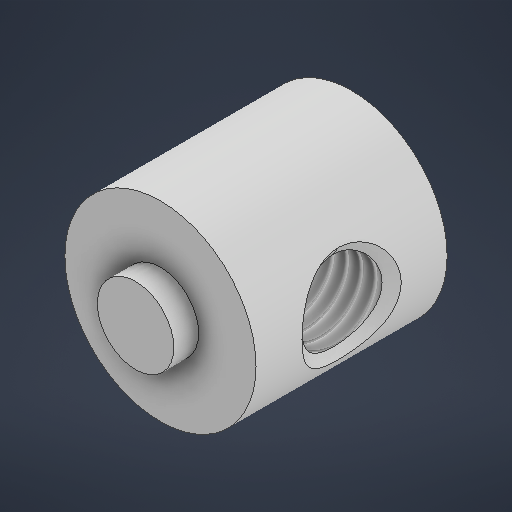
# Autodesk Inventor part: BaseSpacer
Saved by Autodesk Inventor 2025.4 (Build 294407000, 407)
## iProperties
Created: 2026-05-26
Part Number: BaseSpacer
Material: Generic
Document SubType Name: Modeling
Designer: VuQuan
Density: 1 g/cm^3
Appearance: Default
Author: VuQuan
Autodesk Inventor part; units mm, degrees
ref_plane "YZ Plane" through (0, 0, 0) normal (1, 0, 0) x (0, 1, 0)
ref_plane "XZ Plane" through (0, 0, 0) normal (0, 1, 0) x (-1, 0, 0)
ref_plane "XY Plane" through (0, 0, 0) normal (0, 0, 1) x (1, 0, 0)
sketch "Sketch1" plane through (0, 0, 0) normal (0, 0, 1) x (1, 0, 0)
  circle A0 centre (0, 0) radius 10
  circle A1 centre (0, 0) radius 4
  point P0 (-10, 0)
  dimension "d0" = 20
  dimension "d1" = 8
  constraints: 2 coincident, 2 horizontal alignment, 1 centre point, 2 other
  measures "d1" diameter of A1
extrude "Extrusion1" add sketch "Sketch1" along normal mid plane 25.2 contours A1
extrude "Extrusion2" add sketch "Sketch1" along normal mid plane 20
hole "Hole1" at (-10, 0, 0) direction (1, 0, 0) diameter 8.376 end through all thread size "M10x1.5" class "6H" standard "ISO Metric profile"
chamfer "Chamfer1" distance 1 angle 45 8 edges at (9.4815, 3.1784, 2.7271) (9.4815, -3.1783, 2.7272) (9.4815, -3.1784, -2.7271) (9.4815, 3.1783, -2.7272) (-9.4815, 3.1784, 2.7271) (-9.4815, 3.1783, -2.7272) (-9.4815, -3.1784, -2.7271) (-9.4815, -3.1783, 2.7272)
body "Solid1"
